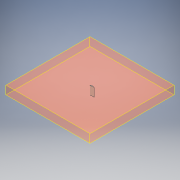
# Autodesk Inventor part: DAE-11
Saved by Autodesk Inventor 2018 (Build 220112000, 112)
## iProperties
Created: 2019-10-30
Part Number: DAE-11
Material: 一般
Document SubType Name: Modeling
Designer: Fluidlab
Density: 1 g/cm^3
Appearance: 既定
Author: Fluidlab
Autodesk Inventor part; units mm, degrees
ref_plane "YZ Plane" through (0, 0, 0) normal (1, 0, 0) x (0, 1, 0)
ref_plane "XZ Plane" through (0, 0, 0) normal (0, 1, 0) x (-1, 0, 0)
ref_plane "XY Plane" through (0, 0, 0) normal (0, 0, 1) x (1, 0, 0)
sketch "スケッチ1" plane through (0, 0, 0) normal (0, 0, 1) x (1, 0, 0)
  spline S0 degree 5 poles (1, 0) (1, 0.0002) (0.9947, 0.0012) (0.9718, 0.0048) (0.9744, 0.0051) (0.9378, 0.0117) (0.9186, 0.0165) (0.8856, 0.0239) (0.8583, 0.031) (0.8275, 0.0392) (0.7977, 0.0476) (0.7671, 0.0564) (0.7367, 0.0654) (0.7059, 0.0747) (0.6758, 0.0836) (0.646, 0.0922) (0.6168, 0.1) (0.588, 0.1071) (0.5594, 0.1131) (0.5308, 0.118) (0.5021, 0.122) (0.4732, 0.1251) (0.4443, 0.1273) (0.4152, 0.1287) (0.3862, 0.1291) (0.3571, 0.1286) (0.3281, 0.1273) (0.2992, 0.125) (0.2705, 0.1219) (0.2421, 0.1179) (0.214, 0.1129) (0.1864, 0.1069) (0.1595, 0.1) (0.1335, 0.0921) (0.1088, 0.0832) (0.0856, 0.0735) (0.0644, 0.0631) (0.0458, 0.0522) (0.0303, 0.0415) (0.0183, 0.0309) (0.0095, 0.0218) (0.004, 0.0132) (0.0008, 0.007) (-0.0003, 0.0007) (0, -0.0031) (0.0019, -0.0068) (0.0048, -0.0095) (0.0097, -0.0115) (0.0172, -0.0132) (0.0294, -0.0146) (0.0466, -0.0152) (0.0692, -0.0152) (0.0953, -0.0145) (0.1241, -0.0133) (0.1545, -0.0118) (0.1858, -0.01) (0.2177, -0.008) (0.2499, -0.0061) (0.2822, -0.0041) (0.3146, -0.0021) (0.3469, -0.0001) (0.3792, 0.0018) (0.4114, 0.0036) (0.4435, 0.0052) (0.4755, 0.0068) (0.5075, 0.0082) (0.5394, 0.0094) (0.5713, 0.0103) (0.6031, 0.0111) (0.6349, 0.0116) (0.6666, 0.0119) (0.6983, 0.012) (0.7301, 0.0118) (0.7617, 0.0115) (0.7935, 0.0108) (0.8246, 0.01) (0.8569, 0.0087) (0.8852, 0.0077) (0.9199, 0.0055) (0.9382, 0.0049) (0.9738, 0.0016) (0.972, 0.0027) (0.9946, 0.0002) (1, -0.0002) (1, 0) knots 0 0 0 0 0 0 0.012125 0.021208 0.033117 0.045961 0.059549 0.073565 0.087659 0.10178 0.115961 0.130172 0.144366 0.158494 0.172505 0.186369 0.200102 0.213741 0.227324 0.240885 0.254446 0.268016 0.281594 0.295176 0.308756 0.322329 0.335888 0.349423 0.362923 0.376372 0.389749 0.40302 0.416144 0.429057 0.441673 0.453862 0.465462 0.476296 0.486196 0.495047 0.502838 0.509565 0.51543 0.520681 0.525642 0.530715 0.53648 0.5434 0.551835 0.561897 0.573459 0.586195 0.599698 0.613617 0.627749 0.641993 0.656299 0.670634 0.684978 0.699317 0.713642 0.727948 0.742236 0.756506 0.770758 0.784995 0.799218 0.81343 0.827634 0.841832 0.856024 0.870211 0.88439 0.898563 0.912738 0.926916 0.940927 0.954453 0.967206 0.978987 0.98793 1 1 1 1 1 1
  point P0 (0, 0)
  point P1 (0.97, 0.0056)
  point P2 (0.9479, 0.01)
  point P3 (0.9186, 0.0164)
  point P4 (0.888, 0.0236)
  point P5 (0.858, 0.0311)
  point P6 (0.828, 0.0392)
  point P7 (0.7978, 0.0476)
  point P8 (0.7674, 0.0564)
  point P9 (0.7366, 0.0655)
  point P10 (0.7057, 0.0747)
  point P11 (0.6752, 0.0837)
  point P12 (0.6454, 0.0922)
  point P13 (0.6163, 0.1)
  point P14 (0.5876, 0.1069)
  point P15 (0.5591, 0.1128)
  point P16 (0.5307, 0.1178)
  point P17 (0.502, 0.1218)
  point P18 (0.4732, 0.1249)
  point P19 (0.4443, 0.1271)
  point P20 (0.4153, 0.1284)
  point P21 (0.3862, 0.1289)
  point P22 (0.3571, 0.1284)
  point P23 (0.3281, 0.127)
  point P24 (0.2991, 0.1248)
  point P25 (0.2704, 0.1217)
  point P26 (0.2419, 0.1176)
  point P27 (0.2138, 0.1126)
  point P28 (0.1861, 0.1066)
  point P29 (0.1591, 0.0995)
  point P30 (0.1329, 0.0915)
  point P31 (0.1079, 0.0825)
  point P32 (0.0844, 0.0726)
  point P33 (0.0629, 0.0618)
  point P34 (0.044, 0.0505)
  point P35 (0.0284, 0.0393)
  point P36 (0.0165, 0.0287)
  point P37 (0.0083, 0.0193)
  point P38 (0.0033, 0.0115)
  point P39 (0.0008, 0.0051)
  point P40 (0, 0)
  point P41 (0.0005, -0.0035)
  point P42 (0.002, -0.0064)
  point P43 (0.0044, -0.0088)
  point P44 (0.0081, -0.0107)
  point P45 (0.0141, -0.0124)
  point P46 (0.0246, -0.0139)
  point P47 (0.0415, -0.0149)
  point P48 (0.0649, -0.0151)
  point P49 (0.0926, -0.0145)
  point P50 (0.1226, -0.0133)
  point P51 (0.1537, -0.0117)
  point P52 (0.1854, -0.01)
  point P53 (0.2174, -0.0081)
  point P54 (0.2497, -0.0061)
  point P55 (0.2822, -0.0041)
  point P56 (0.3146, -0.0021)
  point P57 (0.347, -0.0001)
  point P58 (0.3792, 0.0018)
  point P59 (0.4114, 0.0035)
  point P60 (0.4436, 0.0052)
  point P61 (0.4756, 0.0067)
  point P62 (0.5076, 0.0081)
  point P63 (0.5395, 0.0093)
  point P64 (0.5713, 0.0103)
  point P65 (0.6031, 0.011)
  point P66 (0.6349, 0.0116)
  point P67 (0.6666, 0.0119)
  point P68 (0.6984, 0.0119)
  point P69 (0.7301, 0.0118)
  point P70 (0.7618, 0.0114)
  point P71 (0.7934, 0.0108)
  point P72 (0.825, 0.0099)
  point P73 (0.8566, 0.0088)
  point P74 (0.8883, 0.0073)
  point P75 (0.92, 0.0056)
  point P76 (0.948, 0.0039)
  point P77 (0.9697, 0.0023)
  point P78 (0.9863, 0.0011)
  constraints: 80 other
extrude "押し出し1" add sketch "スケッチ1" along normal blind 2
sketch "スケッチ2" plane through (0, 0, 2) normal (0, 0, 1) x (1, 0, 0)
  line L0 (-10, 10) -> (10, 10)
  line L1 (10, 10) -> (10, -10)
  line L2 (10, -10) -> (-10, -10)
  line L3 (-10, -10) -> (-10, 10)
  line L4 (-10, 10) -> (10, -10) construction
  line L5 (10, 10) -> (-10, -10) construction
  point P0 (0, 0)
  dimension "d2" = 20
  dimension "d3" = 20
  constraints: 12 end point, 2 midpoint, 2 parallel, 1 horizontal, 1 perpendicular
  measures "d2" distance of L1.end L2.end
  measures "d3" distance of L0.end L1.end
surface extrude "押し出しサーフェス1" sketch "スケッチ2" against normal blind 2 shown yes curves L0 L1 L2 L3
sketch "スケッチ3" plane through (-10, 10, 2) normal (0, 1, 0) x (1, 0, 0)
  line L0 (0, 2) -> (20, 2) projected
  line L1 (0, 0) -> (20, 0) projected
  point P0 (10, 2)
surface extrude "押し出しサーフェス2" sketch "スケッチ3" against normal up to surface (20 mm away) shown yes curves L1
sketch "スケッチ4" plane through (-10, 10, 2) normal (0, 1, 0) x (1, 0, 0)
  line L0 (0, 2) -> (20, 2) projected
  point P0 (10, 2)
surface extrude "押し出しサーフェス3" sketch "スケッチ4" against normal up to surface (20 mm away) shown yes curves L0
body "Srf1"
body "Srf2"
body "Srf3"
